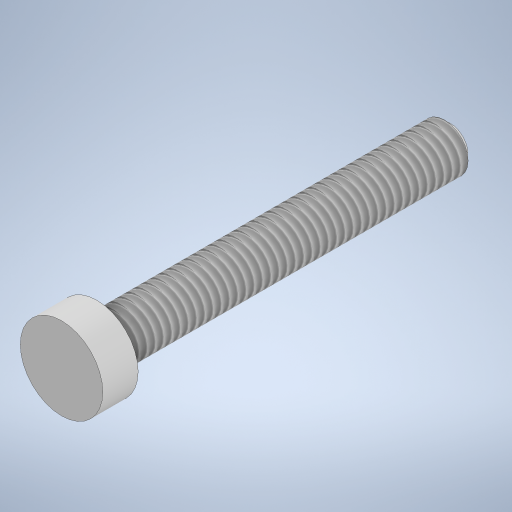
# Autodesk Inventor part: Болт М4х30
Saved by Autodesk Inventor 2023 (Build 270158000, 158)
## iProperties
Created: 2022-05-01
Part Number: Болт М4х30
Material: Типовые
Document SubType Name: Modeling
Designer: User
Density: 1 g/cm^3
Appearance: По умолчанию
Author: User
Autodesk Inventor part; units mm, degrees
ref_plane "YZ Plane" through (0, 0, 0) normal (1, 0, 0) x (0, 1, 0)
ref_plane "XZ Plane" through (0, 0, 0) normal (0, 1, 0) x (-1, 0, 0)
ref_plane "XY Plane" through (0, 0, 0) normal (0, 0, 1) x (1, 0, 0)
sketch "Эскиз1" plane through (0, 0, 0) normal (0, 1, 0) x (-1, 0, 0)
  line L0 (0, 0) -> (3.5, 0)
  line L1 (3.5, 0) -> (3.5, -3)
  line L2 (0, -3) -> (2, -3)
  line L3 (2, -3) -> (2, -33)
  line L4 (2, -33) -> (0, -33)
  line L5 (3.5, -3) -> (2, -3)
  line L6 (0, 0) -> (0, -33)
  dimension "d0" = 3.5
  dimension "d1" = 3
  dimension "d2" = 2
  dimension "d3" = 30
  constraints: 14 end point, 4 perpendicular, 2 horizontal, 1 parallel
  measures "d0" distance of L0.start L0.end
  measures "d1" distance of L0.end L1.end
  measures "d2" distance of L2.start L2.end
  measures "d3" distance of L2.end L3.end
revolve "Вращение1" add sketch "Эскиз1" angle 360 about axis through (0, 0, 0) along (0, 0, -1)
thread "Резьба1" size "M4x0.7" class "6g" standard "ANSI Metric M Profile" full length
chamfer "Фаска1" distance 0.5 angle 45 1 edges at (2, 0, -33)
